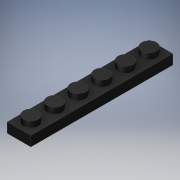
# Autodesk Inventor part: 1x6 short black pegged
Saved by Autodesk Inventor 2017 (Build 210142000, 142)
## iProperties
Created: 2018-05-09
Part Number: 1x6 short black pegged
Material: ABS Plastic
Document SubType Name: Modeling
Designer: Kyle
Density: 1.06 g/cm^3
Appearance: Glossy - Black
Author: Kyle
Autodesk Inventor part; units mm, degrees
ref_plane "YZ Plane" through (0, 0, 0) normal (1, 0, 0) x (0, 1, 0)
ref_plane "XZ Plane" through (0, 0, 0) normal (0, 1, 0) x (-1, 0, 0)
ref_plane "XY Plane" through (0, 0, 0) normal (0, 0, 1) x (1, 0, 0)
sketch "Sketch1" plane through (0, 0, 0) normal (0, 1, 0) x (-1, 0, 0)
  line L0 (0, 0) -> (7.7978, 0)
  line L1 (7.7978, 0) -> (7.7978, -46.7868)
  line L2 (7.7978, -46.7868) -> (0, -46.7868)
  line L3 (0, -46.7868) -> (0, 0)
  dimension "d0" = 7.7978
  dimension "d1" = 46.7868
  constraints: 8 end point, 2 parallel, 1 horizontal, 1 perpendicular
  measures "d0" distance of L1.end L2.end
  measures "d1" distance of L0.end L1.end
extrude "Extrusion1" add sketch "Sketch1" along normal blind 3.236
sketch "Sketch2" plane through (0, 3.236, 0) normal (0, 1, 0) x (1, 0, 0)
  line L0 (0, 0) -> (-3.8989, 0) construction
  line L1 (-3.8989, 0) -> (-3.8989, 3.8989) construction
  line L2 (-3.8989, 3.8989) -> (0, 3.8989) construction
  line L3 (0, 3.8989) -> (0, 0) construction
  circle A0 centre (-3.8989, 3.8989) radius 2.4498
  dimension "d4" = 3.8989
  dimension "d5" = 3.8989
  dimension "d6" = 4.8997
  constraints: 8 end point, 2 parallel, 1 centre point, 1 coincident, 1 horizontal, 1 perpendicular
  measures "d4" distance of L1.end L2.end
  measures "d5" distance of L0.end L1.end
  measures "d6" diameter of A0
extrude "Extrusion2" add sketch "Sketch2" along normal blind 1.9837
pattern_linear "Rectangular Pattern1" count 6 spacing 7.7978 along (0, 0, -1) of "Extrusion2"
shell "Shell1" thickness 1.4732 removed faces 1 at (-2.5993, 0, -15.5956)
sketch "Sketch3" plane through (-6.3246, 1.7628, -1.4732) normal (0, -1, 0) x (1, 0, 0)
  circle A0 centre (2.4257, -2.4257) radius 2.4498 construction
  circle A1 centre (2.4257, -10.2235) radius 2.4498 construction
  line L0 (2.4257, -2.4257) -> (2.4257, -10.2235) construction
  circle A2 centre (2.4257, -6.3246) radius 0.6198
  circle A3 centre (2.4257, -6.3246) radius 1.4491
  point P0 (6.3246, 1.4732)
  dimension "d13" = 1.2395
  constraints: 2 centre point, 2 end point, 1 coincident, 1 midpoint, 1 vertical
  measures "d13" diameter of A2
extrude "Extrusion3" add sketch "Sketch3" along normal up to surface (1.7628 mm away)
pattern_linear "Rectangular Pattern2" count 5 spacing 7.7978 along (0, 0, -1) of "Extrusion3"
body "Solid1"
